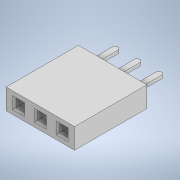
# Autodesk Inventor part: Stiftleiste_3Pin
Saved by Autodesk Inventor 2021 (Build 250183000, 183)
## iProperties
Created: 2024-05-18
Part Number: Stiftleiste_3Pin
Material: Generic
Document SubType Name: Modeling
Designer: Lukas
Density: 1 g/cm^3
Appearance: Default
Author: Lukas
Autodesk Inventor part; units mm, degrees
ref_plane "YZ Plane" through (0, 0, 0) normal (1, 0, 0) x (0, 1, 0)
ref_plane "XZ Plane" through (0, 0, 0) normal (0, 1, 0) x (-1, 0, 0)
ref_plane "XY Plane" through (0, 0, 0) normal (0, 0, 1) x (1, 0, 0)
sketch "Sketch1" plane through (0, 0, 0) normal (0, 0, 1) x (1, 0, 0)
  line L0 (-4, 1.2) -> (4, 1.2)
  line L1 (4, 1.2) -> (4, -1.2)
  line L2 (4, -1.2) -> (-4, -1.2)
  line L3 (-4, -1.2) -> (-4, 1.2)
  line L4 (-3.04, 0.5) -> (-2.04, 0.5)
  line L5 (-2.04, 0.5) -> (-2.04, -0.5)
  line L6 (-2.04, -0.5) -> (-3.04, -0.5)
  line L7 (-3.04, -0.5) -> (-3.04, 0.5)
  line L8 (-0.5, 0.5) -> (0.5, 0.5)
  line L9 (0.5, 0.5) -> (0.5, -0.5)
  line L10 (0.5, -0.5) -> (-0.5, -0.5)
  line L11 (-0.5, -0.5) -> (-0.5, 0.5)
  line L12 (2.04, 0.5) -> (3.04, 0.5)
  line L13 (3.04, 0.5) -> (3.04, -0.5)
  line L14 (3.04, -0.5) -> (2.04, -0.5)
  line L15 (2.04, -0.5) -> (2.04, 0.5)
  point P0 (0, 0)
  point P1 (-4, 0)
  point P2 (0, 1.2)
  point P3 (-2.04, 0)
  point P4 (-0.5, 0)
  point P5 (0, 0.5)
  dimension "d0" = 8
  dimension "d1" = 2.4
  dimension "d2" = 1
  dimension "d3" = 2.54
  dimension "d4" = 2.54
  constraints: 32 end point, 8 parallel, 5 equal length, 5 midpoint, 4 horizontal, 4 perpendicular, 3 horizontal alignment, 2 vertical alignment, 1 point on line
  measures "d0" distance of L0.start L0.end
  measures "d1" distance of L0.end L1.end
  measures "d2" distance of L4.start L4.end
  measures "d3" distance between parallel lines of L9 L5
  measures "d4" distance between parallel lines of L13 L9
extrude "Extrusion1" add sketch "Sketch1" along normal blind 8.45
sketch "Sketch2" plane through (0, 0, 0) normal (0, 0, -1) x (-1, 0, 0)
  line L0 (4, -1.2) -> (-4, -1.2) projected
  line L1 (4, 1.2) -> (4, -1.2) projected
  line L2 (-4, 1.2) -> (4, 1.2) projected
  line L3 (-4, -1.2) -> (-4, 1.2) projected
  line L4 (-2.04, 0.5) -> (-3.04, 0.5) projected
  line L5 (-2.04, -0.5) -> (-2.04, 0.5) projected
  line L6 (-3.04, -0.5) -> (-2.04, -0.5) projected
  line L7 (-3.04, 0.5) -> (-3.04, -0.5) projected
  line L8 (0.5, 0.5) -> (-0.5, 0.5) projected
  line L9 (0.5, -0.5) -> (0.5, 0.5) projected
  line L10 (-0.5, -0.5) -> (0.5, -0.5) projected
  line L11 (-0.5, 0.5) -> (-0.5, -0.5) projected
  line L12 (3.04, 0.5) -> (2.04, 0.5) projected
  line L13 (3.04, -0.5) -> (3.04, 0.5) projected
  line L14 (2.04, -0.5) -> (3.04, -0.5) projected
  line L15 (2.04, 0.5) -> (2.04, -0.5) projected
  point P0 (0, 0)
extrude "Extrusion2" add sketch "Sketch2" against normal blind 1 contours L5 L6 L7 L4 | L9 L10 L11 L8 | L13 L14 L15 L12
sketch "Sketch3" plane through (0, 0, 0) normal (0, 0, -1) x (-1, 0, 0)
  line L0 (-2.865, 0.1875) -> (-2.215, 0.1875)
  line L1 (-2.215, 0.1875) -> (-2.215, -0.1875)
  line L2 (-2.215, -0.1875) -> (-2.865, -0.1875)
  line L3 (-2.865, -0.1875) -> (-2.865, 0.1875)
  line L4 (-0.325, 0.1875) -> (0.325, 0.1875)
  line L5 (0.325, 0.1875) -> (0.325, -0.1875)
  line L6 (0.325, -0.1875) -> (-0.325, -0.1875)
  line L7 (-0.325, -0.1875) -> (-0.325, 0.1875)
  line L8 (2.215, 0.1875) -> (2.865, 0.1875)
  line L9 (2.865, 0.1875) -> (2.865, -0.1875)
  line L10 (2.865, -0.1875) -> (2.215, -0.1875)
  line L11 (2.215, -0.1875) -> (2.215, 0.1875)
  point P0 (0, 0)
  point P1 (0, 0.1875)
  point P2 (-0.325, 0)
  dimension "d9" = 2.54
  dimension "d10" = 2.54
  dimension "d11" = 0.65
  dimension "d12" = 0.375
  constraints: 24 end point, 6 parallel, 3 equal length, 3 horizontal, 3 perpendicular, 3 point on line, 2 midpoint, 1 horizontal alignment, 1 vertical alignment
  measures "d9" distance between parallel lines of L7 L3
  measures "d10" distance between parallel lines of L9 L5
  measures "d11" distance of L4.start L4.end
  measures "d12" distance of L8.end L9.end
extrude "Extrusion3" add sketch "Sketch3" along normal blind 3.15
chamfer "Chamfer1" distance 0.2 angle 45 18 edges at (2.865, 0, -3.15) (2.215, 0, -3.15) (0.325, 0, -3.15) (-0.325, 0, -3.15) (-2.215, 0, -3.15) (-2.865, 0, -3.15) (-2.54, 0.5, 8.45) (-3.04, 0, 8.45) (-2.54, -0.5, 8.45) (-2.04, 0, 8.45) (-0.5, 0, 8.45) (0, 0.5, 8.45) (0.5, 0, 8.45) (0, -0.5, 8.45) (2.04, 0, 8.45) (2.54, 0.5, 8.45) (2.54, -0.5, 8.45) (3.04, 0, 8.45)
equation "\"d4\" = d3"
body "Solid1"
